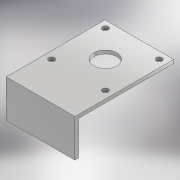
# Autodesk Inventor part: Nema23MountPlate
Saved by Autodesk Inventor 2020.3 (Build 243373000, 373)
## iProperties
Created: 2021-08-24
Part Number: Nema23MountPlate
Material: Aluminum 6061
Document SubType Name: Modeling
Designer: justi
Density: 2.7 g/cm^3
Appearance: Aluminum - Polished
Author: justi
Autodesk Inventor part; units mm, degrees
ref_plane "YZ Plane" through (0, 0, 0) normal (1, 0, 0) x (0, 1, 0)
ref_plane "XZ Plane" through (0, 0, 0) normal (0, 1, 0) x (-1, 0, 0)
ref_plane "XY Plane" through (0, 0, 0) normal (0, 0, 1) x (1, 0, 0)
sketch "Sketch1" plane through (0, 0, 0) normal (0, 0, 1) x (1, 0, 0)
  line L0 (-30, 40) -> (30, 40)
  line L1 (0, 40) -> (0, 10.3) construction
  circle A0 centre (0, 10.3) radius 10
  line L2 (-23.5, -13.2) -> (23.5, -13.2) construction
  line L3 (23.5, -13.2) -> (23.5, 33.8) construction
  line L4 (23.5, 33.8) -> (-23.5, 33.8) construction
  line L5 (-23.5, 33.8) -> (-23.5, -13.2) construction
  line L6 (23.5, -13.2) -> (-23.5, 33.8) construction
  circle A1 centre (-23.5, 33.8) radius 2.55
  circle A2 centre (23.5, 33.8) radius 2.55
  circle A3 centre (-23.5, -13.2) radius 2.55
  circle A4 centre (23.5, -13.2) radius 2.55
  line L7 (0, -46.275) -> (-30, -46.275)
  line L8 (0, -46.275) -> (30, -46.275)
  line L9 (-30, 40) -> (-30, -46.275)
  line L10 (30, 40) -> (30, -46.275)
  point P0 (0, 0)
  dimension "d2" = 29.7
  dimension "d3" = 20
  dimension "d4" = 47
  dimension "d5" = 47
  dimension "d6" = 5.1
  dimension "d7" = 5.1
  dimension "d8" = 5.1
  dimension "d9" = 5.1
  dimension "d12" = 56.575
  dimension "d13" = 30
  dimension "d14" = 30
  constraints: 22 end point, 5 centre point, 5 coincident, 4 horizontal, 3 parallel, 2 midpoint, 2 perpendicular, 1 vertical
  measures "d2" distance of L1.start L1.end
  measures "d3" diameter of A0
  measures "d4" distance of L4.end L3.end
  measures "d5" distance of L3.end L2.end
  measures "d6" diameter of A1
  measures "d7" diameter of A2
  measures "d8" diameter of A3
  measures "d9" diameter of A4
  measures "d12" distance of A0.centre L7.start
  measures "d13" distance of L7.start L7.end
  measures "d14" distance of L7.start L8.end
extrude "Extrusion1" add sketch "Sketch1" along normal blind 3
sketch "Sketch2" plane through (0, 0, 0) normal (0, 0, -1) x (-1, 0, 0)
  line L0 (30, -46.275) -> (-30, -46.275) projected
  line L1 (-30, -46.275) -> (-30, 40) projected
  line L2 (30, -46.275) -> (-30, -46.275)
  line L3 (-30, -46.275) -> (-30, -43.275)
  line L4 (-30, -43.275) -> (30, -43.275)
  line L5 (30, -43.275) -> (30, -46.275)
  point P0 (0, 0)
  dimension "d15" = 3
  constraints: 8 end point, 2 parallel, 1 horizontal, 1 perpendicular, 1 point on line
  measures "d15" distance of L2.end L3.end
extrude "Extrusion2" add sketch "Sketch2" along normal blind 30
body "Solid1"
